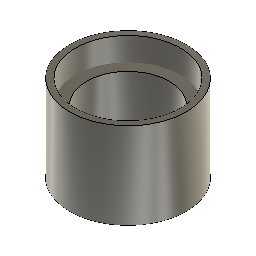
FILAMENTGUIDEadaptor (Autodesk Fusion 360 design; units mm, degrees)
Autodesk Fusion 360 part; units mm, degrees
sketch "Sketch1" plane through (0, 0, 0) normal (0, 0, 1) x (1, 0, 0)
  circle A0 centre (0, 0) radius 5
  dimension "d1" = 10
  constraint coincident A0.centre origin
  measures "d1" diameter of A0
extrude "Extrude1" add sketch "Sketch1" along normal blind 7.4
hole "Hole1" at (0, 0, 7.4) direction (0, 0, -1) diameter 7.1 depth 8 tip angle 118 counterbore diameter 9 counterbore depth 2
